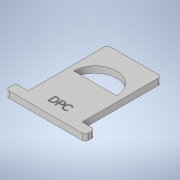
# Autodesk Inventor part: 00_Slider_Mask_DPC
Saved by Autodesk Inventor 2022 (Build 260153000, 153)
## iProperties
Created: 2021-10-22
Part Number: 00_Slider_Mask_DPC
Material: Generic
Document SubType Name: Modeling
Designer: diederichbenedict
Density: 1 g/cm^3
Appearance: Default
Author: diederichbenedict
Autodesk Inventor part; units mm, degrees
ref_plane "YZ Plane" through (0, 0, 0) normal (1, 0, 0) x (0, 1, 0)
ref_plane "XZ Plane" through (0, 0, 0) normal (0, 1, 0) x (-1, 0, 0)
ref_plane "XY Plane" through (0, 0, 0) normal (0, 0, 1) x (1, 0, 0)
sketch "Sketch1" plane through (0, 0, 0) normal (0, 1, 0) x (-1, 0, 0)
  line L0 (-17, 25) -> (17, 25)
  line L1 (17, 25) -> (17, -25)
  line L2 (17, -25) -> (-17, -25)
  line L3 (-17, -25) -> (-17, 25)
  line L4 (-17, 25) -> (17, -25) construction
  line L5 (17, 25) -> (-17, -25) construction
  line L6 (9, -17) -> (9, 17)
  line L7 (9, 17) -> (-9, 17)
  line L8 (-9, 17) -> (-9, -17)
  line L9 (-9, -17) -> (9, -17)
  line L10 (-25, 31) -> (25, 31)
  line L11 (25, 31) -> (25, 25)
  line L12 (25, 25) -> (-25, 25)
  line L13 (-25, 25) -> (-25, 31)
  line L14 (-25, 31) -> (25, 25) construction
  line L15 (25, 31) -> (-25, 25) construction
  point P0 (0, 0)
  point P1 (0, 28)
  point P2 (0, 25)
  dimension "d0" = 34
  dimension "d1" = 50
  dimension "d2" = 8
  dimension "d3" = 50
  dimension "d4" = 6
  constraints: 32 end point, 6 midpoint, 6 parallel, 3 perpendicular, 2 horizontal, 3 other
  measures "d0" distance of L1.end L2.end
  measures "d1" distance of L0.end L1.end
  measures "d2" distance between parallel lines of L1 L6
  measures "d3" distance of L11.end L12.end
  measures "d4" distance of L10.end L11.end
extrude "Extrusion1" add sketch "Sketch1" along normal blind 4 contours L12 L13 L10 L11 L0 | L0 L1 L2 L3 | L9 L8 L7 L6
sketch "Sketch2" plane through (0, 4, 0) normal (0, 1, 0) x (1, 0, 0)
  line L0 (25, -25) -> (17, -25) projected
  line L1 (17, -25) -> (17, 25) projected
  line L2 (17, 25) -> (-17, 25) projected
  line L3 (-17, 25) -> (-17, -25) projected
  line L4 (-17, -25) -> (-25, -25) projected
  line L5 (-25, -25) -> (-25, -31) projected
  line L6 (-25, -31) -> (25, -31) projected
  line L7 (25, -31) -> (25, -25) projected
  line L8 (13.5, 17) -> (-13.5, 17)
  line L9 (-13.5, 17) -> (-13.5, -17)
  line L10 (-13.5, -17) -> (13.5, -17)
  line L11 (13.5, -17) -> (13.5, 17)
  line L12 (13.5, 17) -> (-13.5, -17) construction
  line L13 (-13.5, 17) -> (13.5, -17) construction
  circle A0 centre (0, 0.2783) radius 13.5
  line L14 (-13.5, 0.2783) -> (13.5, 0.2783)
  point P0 (-1.4697, 0.3)
  point P1 (1.4697, 0.3)
  point P2 (13.5, 0)
  point P3 (-13.5, 0)
  dimension "d7" = 27
  dimension "d8" = 34
  constraints: 14 end point, 2 parallel, 2 point on circle, 2 point on line, 1 centre point, 1 horizontal, 1 perpendicular
  measures "d7" distance of L10.end L9.end
  measures "d8" distance of L9.end L8.end
extrude "Extrusion2" cut sketch "Sketch2" against normal through all contours L14 A0 picked at (2.5563, 3.9817)
sketch "Sketch3" plane through (0, 4, 0) normal (0, 1, 0) x (1, 0, 0)
  line L0 (-6.091, -19.1641) -> (19.1348, -19.1641) construction
  line L1 (19.1348, -19.1641) -> (19.1348, -24.3512) construction
  line L2 (19.1348, -24.3512) -> (-6.091, -24.3512) construction
  line L3 (-6.091, -24.3512) -> (-6.091, -19.1641) construction
  spline S0 degree 2 poles (-1.7599, -21.6886) (-1.7599, -22.3553) (-2.3003, -23.4282) (-2.7539, -23.728) knots 0 0 0 1 2 2 2
  spline S1 degree 2 poles (-2.7539, -23.728) (-3.1247, -23.9607) (-3.886, -24.1185) (-4.4777, -24.1185) knots 0 0 0 1 2 2 2
  line L4 (-4.4777, -24.1185) -> (-5.598, -24.1185)
  line L5 (-5.598, -24.1185) -> (-5.598, -19.2508)
  line L6 (-5.598, -19.2508) -> (-4.4895, -19.2508)
  spline S2 degree 2 poles (-4.4895, -19.2508) (-3.8032, -19.2508) (-3.0221, -19.456) (-2.746, -19.6374) knots 0 0 0 1 2 2 2
  spline S3 degree 2 poles (-2.746, -19.6374) (-2.2766, -19.949) (-1.7599, -20.9786) (-1.7599, -21.6886) knots 0 0 0 1 2 2 2
  spline S4 degree 2 poles (-2.4344, -21.6807) (-2.4344, -21.1206) (-2.8052, -20.3277) (-3.172, -20.1029) knots 0 0 0 1 2 2 2
  spline S5 degree 2 poles (-3.172, -20.1029) (-3.4324, -19.949) (-4.0201, -19.811) (-4.458, -19.811) knots 0 0 0 1 2 2 2
  line L7 (-4.458, -19.811) -> (-4.9511, -19.811)
  line L8 (-4.9511, -19.811) -> (-4.9511, -23.5584)
  line L9 (-4.9511, -23.5584) -> (-4.458, -23.5584)
  spline S6 degree 2 poles (-4.458, -23.5584) (-4.028, -23.5584) (-3.3772, -23.4203) (-3.1129, -23.2349) knots 0 0 0 1 2 2 2
  spline S7 degree 2 poles (-3.1129, -23.2349) (-2.7736, -23.0061) (-2.4344, -22.2488) (-2.4344, -21.6807) knots 0 0 0 1 2 2 2
  spline S8 degree 2 poles (2.0191, -20.7182) (2.0191, -21.0338) (1.7942, -21.6018) (1.5931, -21.7991) knots 0 0 0 1 2 2 2
  spline S9 degree 2 poles (1.5931, -21.7991) (1.3406, -22.0476) (0.6582, -22.304) (0.1375, -22.304) knots 0 0 0 1 2 2 2
  line L10 (0.1375, -22.304) -> (-0.4108, -22.304)
  line L11 (-0.4108, -22.304) -> (-0.4108, -24.1185)
  line L12 (-0.4108, -24.1185) -> (-1.0577, -24.1185)
  line L13 (-1.0577, -24.1185) -> (-1.0577, -19.2508)
  line L14 (-1.0577, -19.2508) -> (0.1651, -19.2508)
  spline S10 degree 2 poles (0.1651, -19.2508) (0.599, -19.2508) (1.2065, -19.3929) (1.4392, -19.5546) knots 0 0 0 1 2 2 2
  spline S11 degree 2 poles (1.4392, -19.5546) (1.7114, -19.74) (2.0191, -20.3119) (2.0191, -20.7182) knots 0 0 0 1 2 2 2
  spline S12 degree 2 poles (1.3446, -20.738) (1.3446, -20.4855) (1.171, -20.1147) (0.9935, -19.9964) knots 0 0 0 1 2 2 2
  spline S13 degree 2 poles (0.9935, -19.9964) (0.8396, -19.8938) (0.4294, -19.811) (0.1257, -19.811) knots 0 0 0 1 2 2 2
  line L15 (0.1257, -19.811) -> (-0.4108, -19.811)
  line L16 (-0.4108, -19.811) -> (-0.4108, -21.7517)
  line L17 (-0.4108, -21.7517) -> (0.031, -21.7517)
  spline S14 degree 2 poles (0.031, -21.7517) (0.4255, -21.7517) (0.9106, -21.6255) (1.0684, -21.4598) knots 0 0 0 1 2 2 2
  spline S15 degree 2 poles (1.0684, -21.4598) (1.2144, -21.3139) (1.3446, -20.9707) (1.3446, -20.738) knots 0 0 0 1 2 2 2
  spline S16 degree 2 poles (4.5357, -24.2053) (4.0624, -24.2053) (3.2616, -23.8858) (2.9697, -23.5663) knots 0 0 0 1 2 2 2
  spline S17 degree 2 poles (2.9697, -23.5663) (2.6778, -23.2507) (2.3583, -22.304) (2.3583, -21.6886) knots 0 0 0 1 2 2 2
  spline S18 degree 2 poles (2.3583, -21.6886) (2.3583, -21.0772) (2.6699, -20.1699) (2.9658, -19.8346) knots 0 0 0 1 2 2 2
  spline S19 degree 2 poles (2.9658, -19.8346) (3.2577, -19.5072) (4.0545, -19.1641) (4.5476, -19.1641) knots 0 0 0 1 2 2 2
  spline S20 degree 2 poles (4.5476, -19.1641) (4.7921, -19.1641) (5.2221, -19.2351) (5.4036, -19.2903) knots 0 0 0 1 2 2 2
  spline S21 degree 2 poles (5.4036, -19.2903) (5.5613, -19.3416) (5.8888, -19.4875) (6.0505, -19.5743) knots 0 0 0 1 2 2 2
  line L18 (6.0505, -19.5743) -> (6.0505, -20.3553)
  line L19 (6.0505, -20.3553) -> (5.9992, -20.3553)
  spline S22 degree 2 poles (5.9992, -20.3553) (5.9124, -20.2764) (5.6442, -20.0555) (5.4509, -19.949) knots 0 0 0 1 2 2 2
  spline S23 degree 2 poles (5.4509, -19.949) (5.2655, -19.8465) (4.8276, -19.7163) (4.5436, -19.7163) knots 0 0 0 1 2 2 2
  spline S24 degree 2 poles (4.5436, -19.7163) (4.232, -19.7163) (3.6758, -19.9727) (3.4668, -20.2173) knots 0 0 0 1 2 2 2
  spline S25 degree 2 poles (3.4668, -20.2173) (3.2616, -20.4658) (3.0328, -21.2192) (3.0328, -21.6886) knots 0 0 0 1 2 2 2
  spline S26 degree 2 poles (3.0328, -21.6886) (3.0328, -22.1896) (3.2735, -22.9114) (3.4825, -23.16) knots 0 0 0 1 2 2 2
  spline S27 degree 2 poles (3.4825, -23.16) (3.6877, -23.4006) (4.236, -23.6451) (4.5436, -23.6451) knots 0 0 0 1 2 2 2
  spline S28 degree 2 poles (4.5436, -23.6451) (4.8237, -23.6451) (5.301, -23.5071) (5.4864, -23.4045) knots 0 0 0 1 2 2 2
  spline S29 degree 2 poles (5.4864, -23.4045) (5.6639, -23.302) (5.9282, -23.089) (6.0031, -23.014) knots 0 0 0 1 2 2 2
  line L20 (6.0031, -23.014) -> (6.0505, -23.014)
  line L21 (6.0505, -23.014) -> (6.0505, -23.7872)
  spline S30 degree 2 poles (6.0505, -23.7872) (5.8888, -23.8621) (5.6047, -24.0002) (5.4036, -24.0633) knots 0 0 0 1 2 2 2
  spline S31 degree 2 poles (5.4036, -24.0633) (5.1906, -24.1343) (4.8276, -24.2053) (4.5357, -24.2053) knots 0 0 0 1 2 2 2
  point P0 (0, 0)
  constraints: 2 other
extrude "Extrusion3" cut sketch "Sketch3" against normal blind 1
fillet "Fillet1" radius 2 6 edges at (25, 2, 31) (25, 2, 25) (-25, 2, 31) (-25, 2, 25) (-17, 2, -25) (17, 2, -25)
body "Solid1"
